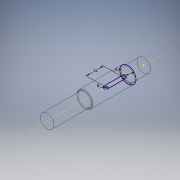
# Autodesk Inventor part: Součást3
Saved by Autodesk Inventor 2019 (Build 230136000, 136)
## iProperties
Created: 2019-10-07
Part Number: Součást3
Material: Všeobecné
Document SubType Name: Modeling
Designer: hynek
Density: 1 g/cm^3
Appearance: Výchozí
Author: hynek
Autodesk Inventor part; units mm, degrees
ref_plane "YZ Plane" through (0, 0, 0) normal (1, 0, 0) x (0, 1, 0)
ref_plane "XZ Plane" through (0, 0, 0) normal (0, 1, 0) x (-1, 0, 0)
ref_plane "XY Plane" through (0, 0, 0) normal (0, 0, 1) x (1, 0, 0)
sketch "Náčrt1" plane through (0, 0, 0) normal (0, 0, 1) x (1, 0, 0)
  circle A0 centre (0, 0) radius 12.5
  dimension "d0" = 25
  constraints: 1 centre point, 1 coincident
  measures "d0" diameter of A0
extrude "Vysunutí1" add sketch "Náčrt1" along normal blind 30
sketch "Náčrt2" plane through (0, 0, 30) normal (0, 0, 1) x (1, 0, 0)
  circle A0 centre (0, 0) radius 15
  dimension "d3" = 30
  constraints: 1 centre point, 1 coincident
  measures "d3" diameter of A0
extrude "Vysunutí2" add sketch "Náčrt2" along normal blind 80
sketch "Náčrt3" plane through (0, 0, 110) normal (0, 0, 1) x (1, 0, 0)
  circle A0 centre (0, 0) radius 12.5
  dimension "d6" = 25
  constraints: 1 centre point, 1 coincident
  measures "d6" diameter of A0
extrude "Vysunutí3" add sketch "Náčrt3" along normal blind 70
sketch "Náčrt4" plane through (0, 0, 0) normal (1, 0, 0) x (0, 1, 0)
  point P0 (0, 0)
sketch "Náčrt5" plane through (0, 0, 0) normal (0, 1, 0) x (-1, 0, 0)
  line L0 (0, -36) -> (0, 216) construction
  arc A0 (-4, 38.6) -> (4, 38.6) centre (0, 38.6) ccw
  line L1 (-15, 30) -> (15, 30) construction
  arc A1 (4, 70.6) -> (-4, 70.6) centre (0, 70.6) ccw
  line L2 (4, 70.6) -> (4, 38.6)
  line L3 (-4, 70.6) -> (-4, 38.6)
  point P0 (0, 0)
  dimension "d9" = 8
  dimension "d10" = 8.6
  dimension "d11" = 8
  dimension "d12" = 32
  constraints: 4 end point, 4 point on circle, 3 tangent, 2 centre point, 2 point on line, 1 vertical
  measures "d9" diameter of A0
  measures "d10" distance from line of L1 A0.centre
  measures "d11" diameter of A1
  measures "d12" distance of A0.centre A1.centre
